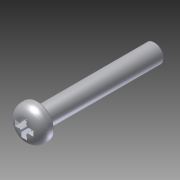
# Autodesk Inventor part: M2.5x16
Saved by Autodesk Inventor 2011 SP1 (Build 150282100, 282)
## iProperties
Created: 2013-12-24
Part Number: M2.5x16
Catalog Web Link: www.cadenas.de
Description: Screw M2.5x16-Screw M2.5x16
Vendor: NKKSWITCHES
Document SubType Name: Modeling
Designer: PARTuser1
Manufacturer: NKKSWITCHES
Density: 1 g/cm^3
Category: PARTsolutions
Company: NKKSWITCHES
Title: M2.5x16
Author: Cadenas PARTsolutions
Comments: Screw M2.5x16
PSOL_IDENT_0: {$CADENAS_DATA\23d-libs\nkkswitches\toggle\s\parts\screw_m2.5x16.prj},163 {VTYP=3D},{NB=M2.5x16},{LI
PSOL_IDENT_1: NA=M2.5x16},{NN=Screw M2.5x16},{DATE=05.04.2013 11:54:55},{GEOMDATE=05.04.2013 13:54:00},{VERSION=},
PSOL_IDENT_2: {LINEID=10},{LINESUBID=-1},{WBVAR=}  {NB=M2.5x16},{LINA=M2.5x16},{KT=DUMMY},{PN=M2.5x16},{D=2.5},{L=
PSOL_IDENT_3: 16.0}
CNS_NN: Screw M2.5x16
CNS_NT: Screw M2.5x16
CNS_NB: M2.5x16
CNS_NBSYN: $PN.
CNS_LINA: M2.5x16
CNS_PN: M2.5x16
CNS_D: 2.5
CNS_L: 16.0
SUPPLIER: NKKSWITCHES
ARTICLENO: M2.5x16
BOMINFO: M2.5x16
CREATOR: CADENAS GmbH
Autodesk Inventor part; units mm, degrees
sketch "Sketch_1" plane through (0, 0, 0) normal (1, 0, 0) x (0, 1, 0)
  line L0 (0, -16) -> (0, 1.905)
  line L1 (0, 1.905) -> (1.016, 1.905)
  arc A0 (2.286, 0.635) -> (1.016, 1.905) centre (1.016, 0.635) ccw
  line L2 (2.286, 0.635) -> (2.286, 0.25)
  arc A1 (2.036, 0) -> (2.286, 0.25) centre (2.036, 0.25) ccw
  line L3 (2.036, 0) -> (1.25, 0)
  line L4 (1.25, 0) -> (1.25, -15.724)
  line L5 (1.25, -15.724) -> (0.974, -16)
  line L6 (0.974, -16) -> (0, -16)
  line L7 (0, -16) -> (0, 1.905)
  constraints: 16 end point, 4 point on circle, 2 centre point
revolve "Revolution1" add sketch "Sketch_1" angle 360 about axis through (0, 0, -16) along (0, 0, -1)
sketch "Sketch_2" plane through (0, 0, 0.508) normal (0, 0, 1) x (1, 0, 0)
  line L0 (-1.25, 0.4) -> (-1.25, -0.4)
  line L1 (-1.25, -0.4) -> (-0.5941, -0.3311)
  line L2 (-0.5941, -0.3311) -> (-0.422, -0.422)
  line L3 (-0.422, -0.422) -> (-0.3311, -0.5941)
  line L4 (-0.3311, -0.5941) -> (-0.4, -1.25)
  line L5 (-0.4, -1.25) -> (0.4, -1.25)
  line L6 (0.4, -1.25) -> (0.3311, -0.5941)
  line L7 (0.3311, -0.5941) -> (0.422, -0.422)
  line L8 (0.422, -0.422) -> (0.5941, -0.3311)
  line L9 (0.5941, -0.3311) -> (1.25, -0.4)
  line L10 (1.25, -0.4) -> (1.25, 0.4)
  line L11 (1.25, 0.4) -> (0.5941, 0.3311)
  line L12 (0.5941, 0.3311) -> (0.422, 0.422)
  line L13 (0.422, 0.422) -> (0.3311, 0.5941)
  line L14 (0.3311, 0.5941) -> (0.4, 1.25)
  line L15 (0.4, 1.25) -> (-0.4, 1.25)
  line L16 (-0.4, 1.25) -> (-0.3311, 0.5941)
  line L17 (-0.3311, 0.5941) -> (-0.422, 0.422)
  line L18 (-0.422, 0.422) -> (-0.5941, 0.3311)
  line L19 (-0.5941, 0.3311) -> (-1.25, 0.4)
  constraints: 40 end point
extrude "Extrusion1" cut sketch "Sketch_2" along normal blind 1.524
ref_plane "IP1_XY" through (0, 0, 0) normal (0, 0, -1) x (1, 0, 0)
ref_plane "IP1_YZ" through (0, 0, 0) normal (1, 0, 0) x (0, -1, 0)
ref_plane "IP1_ZX" through (0, 0, 0) normal (0, -1, 0) x (0, 0, -1)
ref_plane "IP3_XY" through (0, 0, -16) normal (0, 0, -1) x (0, 1, 0)
ref_plane "IP3_YZ" through (0, 0, -16) normal (0, 1, 0) x (1, 0, 0)
ref_plane "IP3_ZX" through (0, 0, -16) normal (1, 0, 0) x (0, 0, -1)
body "Solid1"
